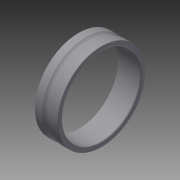
# Autodesk Inventor part: A-1510_ir
Saved by Autodesk Inventor 2014 SP2 (Build 180246200, 246)
## iProperties
Created: 2019-11-12
Part Number: A-1510_ir
Material: Generic
Catalog Web Link: www.cadenas.de
Description: Radial Ball Bearings (A series)  OT ir-Radial Ball Bearings (A series)  Open Type
Vendor: NMB
Document SubType Name: Modeling
Designer: psadmin
Manufacturer: NMB
Mass: 0.0582621 g
Surface Area: 2.37636 cm^2
Volume: 0.0582621 cm^3
Density: 1 g/cm^3
Appearance: PSOLRGB-192-192-192
Category: PARTsolutions
Company: NMB
Title: A-1510_ir
Author: Cadenas PARTsolutions
Comments: Radial Ball Bearings (A series)  Open Type
PSOL_IDENT_0: {$CADENAS_DATA\23d-libs\nmb\pbbp\radial_ball_bear_thin_secti\rbb_as\as_open_ir.prj},191 {VTYP=3D},{N
PSOL_IDENT_1: B=A-1510_ir},{LINA=A-1510_ir},{NN=Radial Ball Bearings (A series)  OT ir},{DATE=11.11.2013 05:13:38}
PSOL_IDENT_2: ,{GEOMDATE=29.10.2013 14:08:00},{VERSION=},{LINEID=860},{WBVAR=},{WBNUMERIC=}  {NB=A-1510_ir},{LINA=
PSOL_IDENT_3: A-1510_ir},{KT=DUMMY},{IDNR=},{PN=A-1510},{SHLD=open},{FLANG=unflanged},{SD=10.000},{D=15.000},{B=3.
PSOL_IDENT_4: 000},{SR=0.15},{BCZ=11},{DW=1.5875},{LI=11.25},{LO=13.63},{D1=0.000},{C1=0.00},{D2=0.0},{C2=0.00},{C
PSOL_IDENT_5: OR=435},{CR=1084},{PCD=12.500},{U=14.088},{W=10.913},{Y=0.794},{Z=0.794},{AA=0.000},{AC=0.00},{AD=0.
PSOL_IDENT_6: 000},{AF=0.00},{AQ=0.00},{AH=0.00},{AI=0.00},{AJ=0.00}
NN: Radial Ball Bearings (A series)  OT ir
NT: Radial Ball Bearings (A series)  Open Type
NB: A-1510_ir
NBSYN: $PN._ir
LINA: A-1510_ir
PN: A-1510
SHLD: open
FLANG: unflanged
SD: 10
D: 15
B: 3
SR: 0.15
BCZ: 11
DW: 1.5875
LI: 11.25
LO: 13.63
D1: 0
C1: 0
D2: 0
C2: 0
COR: 435
CR: 1084
PCD: 12.5
U: 14.088
W: 10.913
Y: 0.794
Z: 0.794
AA: 0
AC: 0
AD: 0
AF: 0
AQ: 0
AH: 0
AI: 0
AJ: 0
SUPPLIER: NMB
ARTICLENO: A-1510_ir
BOMINFO: A-1510_ir
CREATOR: CADENAS GmbH
Autodesk Inventor part; units mm, degrees
sketch "Sketch_1" plane through (0, 0, 0) normal (0, 0, 1) x (1, 0, 0)
  line L0 (3, 0) -> (0, 0)
  line L1 (0, 5.55) -> (0, 5.15)
  arc A0 (0, 5.15) -> (0.15, 5) centre (0.15, 5.15) ccw
  line L2 (0.15, 5) -> (2.85, 5)
  arc A1 (2.85, 5) -> (3, 5.15) centre (2.85, 5.15) ccw
  line L3 (3, 5.15) -> (3, 5.55)
  arc A2 (3, 5.55) -> (2.925, 5.625) centre (2.925, 5.55) ccw
  line L4 (2.925, 5.625) -> (1.9893, 5.625)
  arc A3 (1.0107, 5.625) -> (1.9893, 5.625) centre (1.5, 6.25) ccw
  line L5 (1.0107, 5.625) -> (0.075, 5.625)
  arc A4 (0.075, 5.625) -> (0, 5.55) centre (0.075, 5.55) ccw
  constraints: 12 end point, 10 point on circle, 5 centre point
revolve "Revolution1" add sketch "Sketch_1" angle 360 about axis through (3, 0, 0) along (1, 0, 0)
ref_plane "1_XY" through (1.5, 0, 0) normal (1, 0, 0) x (0, 0, -1)
ref_plane "1_YZ" through (1.5, 0, 0) normal (0, 0, -1) x (0, 1, 0)
ref_plane "1_ZX" through (1.5, 0, 0) normal (0, 1, 0) x (1, 0, 0)
ref_plane "1_Dummy_XY" through (0, 0, 0) normal (-1, 0, 0) x (0, 0, -1)
ref_plane "1_Dummy_YZ" through (0, 0, 0) normal (0, 0, -1) x (0, -1, 0)
ref_plane "1_Dummy_ZX" through (0, 0, 0) normal (0, -1, 0) x (-1, 0, 0)
body "Solid1"
